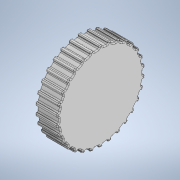
# Autodesk Inventor part: Dial_Main-Sub Menu Dial
Saved by Autodesk Inventor 2021 (Build 250183000, 183)
## iProperties
Created: 2021-05-07
Part Number: Dial_Main-Sub Menu Dial
Material: Generic
Document SubType Name: Modeling
Designer: trent
Density: 1 g/cm^3
Appearance: Default
Author: trent
Autodesk Inventor part; units mm, degrees
ref_plane "YZ Plane" through (0, 0, 0) normal (1, 0, 0) x (0, 1, 0)
ref_plane "XZ Plane" through (0, 0, 0) normal (0, 1, 0) x (-1, 0, 0)
ref_plane "XY Plane" through (0, 0, 0) normal (0, 0, 1) x (1, 0, 0)
sketch "Sketch1" plane through (0, 0, 0) normal (1, 0, 0) x (0, 1, 0)
  arc A0 (9.9984, -0.1796) -> (9.9984, 0.1796) centre (0, 0) ccw
  line L0 (0, 0) -> (11.5, 0)
  line L1 (9.7343, -0.3749) -> (9.7949, -0.376)
  line L2 (9.7343, 0.3749) -> (9.7949, 0.376)
  arc A1 (9.4805, 0.6089) -> (9.7343, 0.3749) centre (9.73, 0.6249) ccw
  arc A2 (9.7343, -0.3749) -> (9.4805, -0.6089) centre (9.73, -0.6249) ccw
  arc A3 (9.9984, 0.1796) -> (9.7949, 0.376) centre (9.7984, 0.176) ccw
  arc A4 (9.7949, -0.376) -> (9.9984, -0.1796) centre (9.7984, -0.176) ccw
  arc A5 (9.8172, 1.9031) -> (9.7426, 2.2545) centre (0, 0) ccw
  line L3 (9.5996, 1.6571) -> (9.6591, 1.6687)
  line L4 (9.4436, 2.3906) -> (9.5027, 2.4042)
  arc A6 (9.7426, 2.2545) -> (9.5027, 2.4042) centre (9.5477, 2.2094) ccw
  arc A7 (9.6591, 1.6687) -> (9.8172, 1.9031) centre (9.6209, 1.865) ccw
  arc A8 (9.1467, 2.5667) -> (9.4436, 2.3906) centre (9.3874, 2.6342) ccw
  arc A9 (9.5996, 1.6571) -> (9.3999, 1.3755) centre (9.6473, 1.4117) ccw
  arc A10 (9.207, 3.9026) -> (9.0609, 4.2308) centre (0, 0) ccw
  line L5 (9.0452, 3.6168) -> (9.101, 3.6405)
  line L6 (8.7402, 4.3018) -> (8.7952, 4.3274)
  arc A11 (9.0609, 4.2308) -> (8.7952, 4.3274) centre (8.8797, 4.1462) ccw
  arc A12 (9.101, 3.6405) -> (9.207, 3.9026) centre (9.0229, 3.8246) ccw
  arc A13 (8.4132, 4.4123) -> (8.7402, 4.3018) centre (8.6346, 4.5284) ccw
  arc A14 (9.0452, 3.6168) -> (8.9085, 3.2998) centre (9.1429, 3.3867) ccw
  arc A15 (8.1944, 5.7316) -> (7.9833, 6.0222) centre (0, 0) ccw
  line L7 (8.0956, 5.4184) -> (8.1453, 5.4531)
  line L8 (7.6549, 6.025) -> (7.7033, 6.0615)
  arc A16 (7.9833, 6.0222) -> (7.7033, 6.0615) centre (7.8236, 5.9018) ccw
  arc A17 (8.1453, 5.4531) -> (8.1944, 5.7316) centre (8.0305, 5.617) ccw
  arc A18 (7.312, 6.0651) -> (7.6549, 6.025) centre (7.5044, 6.2247) ccw
  arc A19 (8.0956, 5.4184) -> (8.0277, 5.0799) centre (8.239, 5.2136) ccw
  arc A20 (6.8237, 7.3101) -> (6.5568, 7.5504) centre (0, 0) ccw
  line L9 (6.7922, 6.9831) -> (6.8335, 7.0275)
  line L10 (6.2349, 7.4849) -> (6.2747, 7.5306)
  arc A21 (6.5568, 7.5504) -> (6.2747, 7.5306) centre (6.4256, 7.3994) ccw
  arc A22 (6.8335, 7.0275) -> (6.8237, 7.3101) centre (6.6872, 7.1639) ccw
  arc A23 (5.8912, 7.4528) -> (6.2349, 7.4849) centre (6.0462, 7.6489) ccw
  arc A24 (6.7922, 6.9831) -> (6.7961, 6.638) centre (6.975, 6.8126) ccw
  arc A25 (5.1547, 8.5691) -> (4.8436, 8.7487) centre (0, 0) ccw
  line L11 (5.1919, 8.2427) -> (5.2231, 8.2947)
  line L12 (4.5425, 8.6176) -> (4.5719, 8.6706)
  arc A26 (4.8436, 8.7487) -> (4.5719, 8.6706) centre (4.7468, 8.5737) ccw
  arc A27 (5.2231, 8.2947) -> (5.1547, 8.5691) centre (5.0516, 8.3977) ccw
  arc A28 (4.2129, 8.5148) -> (4.5425, 8.6176) centre (4.3238, 8.7388) ccw
  arc A29 (5.1919, 8.2427) -> (5.2675, 7.9059) centre (5.4061, 8.1139) ccw
  arc A30 (3.2605, 9.4535) -> (2.9189, 9.5645) centre (0, 0) ccw
  line L13 (3.3646, 9.142) -> (3.3844, 9.1993)
  line L14 (2.6515, 9.3737) -> (2.6692, 9.4317)
  arc A31 (2.9189, 9.5645) -> (2.6692, 9.4317) centre (2.8605, 9.3732) ccw
  arc A32 (3.3844, 9.1993) -> (3.2605, 9.4535) centre (3.1953, 9.2645) ccw
  arc A33 (2.3506, 9.2046) -> (2.6515, 9.3737) centre (2.4124, 9.4468) ccw
  arc A34 (3.3646, 9.142) -> (3.5087, 8.8283) centre (3.601, 9.0606) ccw
  arc A35 (1.2237, 9.9248) -> (0.8665, 9.9624) centre (0, 0) ccw
  line L15 (1.3904, 9.6418) -> (1.3978, 9.702)
  line L16 (0.6446, 9.7202) -> (0.6499, 9.7806)
  arc A36 (0.8665, 9.9624) -> (0.6499, 9.7806) centre (0.8492, 9.7631) ccw
  arc A37 (1.3978, 9.702) -> (1.2237, 9.9248) centre (1.1993, 9.7263) ccw
  arc A38 (0.3854, 9.4922) -> (0.6446, 9.7202) centre (0.3956, 9.742) ccw
  arc A39 (1.3904, 9.6418) -> (1.5965, 9.3649) centre (1.6385, 9.6113) ccw
  arc A40 (-0.8665, 9.9624) -> (-1.2237, 9.9248) centre (0, 0) ccw
  line L17 (-0.6446, 9.7202) -> (-0.6499, 9.7806)
  line L18 (-1.3904, 9.6418) -> (-1.3978, 9.702)
  arc A41 (-1.2237, 9.9248) -> (-1.3978, 9.702) centre (-1.1993, 9.7263) ccw
  arc A42 (-0.6499, 9.7806) -> (-0.8665, 9.9624) centre (-0.8492, 9.7631) ccw
  arc A43 (-1.5965, 9.3649) -> (-1.3904, 9.6418) centre (-1.6385, 9.6113) ccw
  arc A44 (-0.6446, 9.7202) -> (-0.3854, 9.4922) centre (-0.3956, 9.742) ccw
  arc A45 (-2.9189, 9.5645) -> (-3.2605, 9.4535) centre (0, 0) ccw
  line L19 (-2.6515, 9.3737) -> (-2.6692, 9.4317)
  line L20 (-3.3646, 9.142) -> (-3.3844, 9.1993)
  arc A46 (-3.2605, 9.4535) -> (-3.3844, 9.1993) centre (-3.1953, 9.2645) ccw
  arc A47 (-2.6692, 9.4317) -> (-2.9189, 9.5645) centre (-2.8605, 9.3732) ccw
  arc A48 (-3.5087, 8.8283) -> (-3.3646, 9.142) centre (-3.601, 9.0606) ccw
  arc A49 (-2.6515, 9.3737) -> (-2.3506, 9.2046) centre (-2.4124, 9.4468) ccw
  arc A50 (-4.8436, 8.7487) -> (-5.1547, 8.5691) centre (0, 0) ccw
  line L21 (-4.5425, 8.6176) -> (-4.5719, 8.6706)
  line L22 (-5.1919, 8.2427) -> (-5.2231, 8.2947)
  arc A51 (-5.1547, 8.5691) -> (-5.2231, 8.2947) centre (-5.0516, 8.3977) ccw
  arc A52 (-4.5719, 8.6706) -> (-4.8436, 8.7487) centre (-4.7468, 8.5737) ccw
  arc A53 (-5.2675, 7.9059) -> (-5.1919, 8.2427) centre (-5.4061, 8.1139) ccw
  arc A54 (-4.5425, 8.6176) -> (-4.2129, 8.5148) centre (-4.3238, 8.7388) ccw
  arc A55 (-6.5568, 7.5504) -> (-6.8237, 7.3101) centre (0, 0) ccw
  line L23 (-6.2349, 7.4849) -> (-6.2747, 7.5306)
  line L24 (-6.7922, 6.9831) -> (-6.8335, 7.0275)
  arc A56 (-6.8237, 7.3101) -> (-6.8335, 7.0275) centre (-6.6872, 7.1639) ccw
  arc A57 (-6.2747, 7.5306) -> (-6.5568, 7.5504) centre (-6.4256, 7.3994) ccw
  arc A58 (-6.7961, 6.638) -> (-6.7922, 6.9831) centre (-6.975, 6.8126) ccw
  arc A59 (-6.2349, 7.4849) -> (-5.8912, 7.4528) centre (-6.0462, 7.6489) ccw
  arc A60 (-7.9833, 6.0222) -> (-8.1944, 5.7316) centre (0, 0) ccw
  line L25 (-7.6549, 6.025) -> (-7.7033, 6.0615)
  line L26 (-8.0956, 5.4184) -> (-8.1453, 5.4531)
  arc A61 (-8.1944, 5.7316) -> (-8.1453, 5.4531) centre (-8.0305, 5.617) ccw
  arc A62 (-7.7033, 6.0615) -> (-7.9833, 6.0222) centre (-7.8236, 5.9018) ccw
  arc A63 (-8.0277, 5.0799) -> (-8.0956, 5.4184) centre (-8.239, 5.2136) ccw
  arc A64 (-7.6549, 6.025) -> (-7.312, 6.0651) centre (-7.5044, 6.2247) ccw
  arc A65 (-9.0609, 4.2308) -> (-9.207, 3.9026) centre (0, 0) ccw
  line L27 (-8.7402, 4.3018) -> (-8.7952, 4.3274)
  line L28 (-9.0452, 3.6168) -> (-9.101, 3.6405)
  arc A66 (-9.207, 3.9026) -> (-9.101, 3.6405) centre (-9.0229, 3.8246) ccw
  arc A67 (-8.7952, 4.3274) -> (-9.0609, 4.2308) centre (-8.8797, 4.1462) ccw
  arc A68 (-8.9085, 3.2998) -> (-9.0452, 3.6168) centre (-9.1429, 3.3867) ccw
  arc A69 (-8.7402, 4.3018) -> (-8.4132, 4.4123) centre (-8.6346, 4.5284) ccw
  arc A70 (-9.7426, 2.2545) -> (-9.8172, 1.9031) centre (0, 0) ccw
  line L29 (-9.4436, 2.3906) -> (-9.5027, 2.4042)
  line L30 (-9.5996, 1.6571) -> (-9.6591, 1.6687)
  arc A71 (-9.8172, 1.9031) -> (-9.6591, 1.6687) centre (-9.6209, 1.865) ccw
  arc A72 (-9.5027, 2.4042) -> (-9.7426, 2.2545) centre (-9.5477, 2.2094) ccw
  arc A73 (-9.3999, 1.3755) -> (-9.5996, 1.6571) centre (-9.6473, 1.4117) ccw
  arc A74 (-9.4436, 2.3906) -> (-9.1467, 2.5667) centre (-9.3874, 2.6342) ccw
  arc A75 (-9.9984, 0.1796) -> (-9.9984, -0.1796) centre (0, 0) ccw
  line L31 (-9.7343, 0.3749) -> (-9.7949, 0.376)
  line L32 (-9.7343, -0.3749) -> (-9.7949, -0.376)
  arc A76 (-9.9984, -0.1796) -> (-9.7949, -0.376) centre (-9.7984, -0.176) ccw
  arc A77 (-9.7949, 0.376) -> (-9.9984, 0.1796) centre (-9.7984, 0.176) ccw
  arc A78 (-9.4805, -0.6089) -> (-9.7343, -0.3749) centre (-9.73, -0.6249) ccw
  arc A79 (-9.7343, 0.3749) -> (-9.4805, 0.6089) centre (-9.73, 0.6249) ccw
  arc A80 (-9.8172, -1.9031) -> (-9.7426, -2.2545) centre (0, 0) ccw
  line L33 (-9.5996, -1.6571) -> (-9.6591, -1.6687)
  line L34 (-9.4436, -2.3906) -> (-9.5027, -2.4042)
  arc A81 (-9.7426, -2.2545) -> (-9.5027, -2.4042) centre (-9.5477, -2.2094) ccw
  arc A82 (-9.6591, -1.6687) -> (-9.8172, -1.9031) centre (-9.6209, -1.865) ccw
  arc A83 (-9.1467, -2.5667) -> (-9.4436, -2.3906) centre (-9.3874, -2.6342) ccw
  arc A84 (-9.5996, -1.6571) -> (-9.3999, -1.3755) centre (-9.6473, -1.4117) ccw
  arc A85 (-9.207, -3.9026) -> (-9.0609, -4.2308) centre (0, 0) ccw
  line L35 (-9.0452, -3.6168) -> (-9.101, -3.6405)
  line L36 (-8.7402, -4.3018) -> (-8.7952, -4.3274)
  arc A86 (-9.0609, -4.2308) -> (-8.7952, -4.3274) centre (-8.8797, -4.1462) ccw
  arc A87 (-9.101, -3.6405) -> (-9.207, -3.9026) centre (-9.0229, -3.8246) ccw
  arc A88 (-8.4132, -4.4123) -> (-8.7402, -4.3018) centre (-8.6346, -4.5284) ccw
  arc A89 (-9.0452, -3.6168) -> (-8.9085, -3.2998) centre (-9.1429, -3.3867) ccw
  arc A90 (-8.1944, -5.7316) -> (-7.9833, -6.0222) centre (0, 0) ccw
  line L37 (-8.0956, -5.4184) -> (-8.1453, -5.4531)
  line L38 (-7.6549, -6.025) -> (-7.7033, -6.0615)
  arc A91 (-7.9833, -6.0222) -> (-7.7033, -6.0615) centre (-7.8236, -5.9018) ccw
  arc A92 (-8.1453, -5.4531) -> (-8.1944, -5.7316) centre (-8.0305, -5.617) ccw
  arc A93 (-7.312, -6.0651) -> (-7.6549, -6.025) centre (-7.5044, -6.2247) ccw
  arc A94 (-8.0956, -5.4184) -> (-8.0277, -5.0799) centre (-8.239, -5.2136) ccw
  arc A95 (-6.8237, -7.3101) -> (-6.5568, -7.5504) centre (0, 0) ccw
  line L39 (-6.7922, -6.9831) -> (-6.8335, -7.0275)
  line L40 (-6.2349, -7.4849) -> (-6.2747, -7.5306)
  arc A96 (-6.5568, -7.5504) -> (-6.2747, -7.5306) centre (-6.4256, -7.3994) ccw
  arc A97 (-6.8335, -7.0275) -> (-6.8237, -7.3101) centre (-6.6872, -7.1639) ccw
  arc A98 (-5.8912, -7.4528) -> (-6.2349, -7.4849) centre (-6.0462, -7.6489) ccw
  arc A99 (-6.7922, -6.9831) -> (-6.7961, -6.638) centre (-6.975, -6.8126) ccw
  arc A100 (-5.1547, -8.5691) -> (-4.8436, -8.7487) centre (0, 0) ccw
  line L41 (-5.1919, -8.2427) -> (-5.2231, -8.2947)
  line L42 (-4.5425, -8.6176) -> (-4.5719, -8.6706)
  arc A101 (-4.8436, -8.7487) -> (-4.5719, -8.6706) centre (-4.7468, -8.5737) ccw
  arc A102 (-5.2231, -8.2947) -> (-5.1547, -8.5691) centre (-5.0516, -8.3977) ccw
  arc A103 (-4.2129, -8.5148) -> (-4.5425, -8.6176) centre (-4.3238, -8.7388) ccw
  arc A104 (-5.1919, -8.2427) -> (-5.2675, -7.9059) centre (-5.4061, -8.1139) ccw
  arc A105 (-3.2605, -9.4535) -> (-2.9189, -9.5645) centre (0, 0) ccw
  line L43 (-3.3646, -9.142) -> (-3.3844, -9.1993)
  line L44 (-2.6515, -9.3737) -> (-2.6692, -9.4317)
  arc A106 (-2.9189, -9.5645) -> (-2.6692, -9.4317) centre (-2.8605, -9.3732) ccw
  arc A107 (-3.3844, -9.1993) -> (-3.2605, -9.4535) centre (-3.1953, -9.2645) ccw
  arc A108 (-2.3506, -9.2046) -> (-2.6515, -9.3737) centre (-2.4124, -9.4468) ccw
  arc A109 (-3.3646, -9.142) -> (-3.5087, -8.8283) centre (-3.601, -9.0606) ccw
  arc A110 (-1.2237, -9.9248) -> (-0.8665, -9.9624) centre (0, 0) ccw
  line L45 (-1.3904, -9.6418) -> (-1.3978, -9.702)
  line L46 (-0.6446, -9.7202) -> (-0.6499, -9.7806)
  arc A111 (-0.8665, -9.9624) -> (-0.6499, -9.7806) centre (-0.8492, -9.7631) ccw
  arc A112 (-1.3978, -9.702) -> (-1.2237, -9.9248) centre (-1.1993, -9.7263) ccw
  arc A113 (-0.3854, -9.4922) -> (-0.6446, -9.7202) centre (-0.3956, -9.742) ccw
  arc A114 (-1.3904, -9.6418) -> (-1.5965, -9.3649) centre (-1.6385, -9.6113) ccw
  arc A115 (0.8665, -9.9624) -> (1.2237, -9.9248) centre (0, 0) ccw
  line L47 (0.6446, -9.7202) -> (0.6499, -9.7806)
  line L48 (1.3904, -9.6418) -> (1.3978, -9.702)
  arc A116 (1.2237, -9.9248) -> (1.3978, -9.702) centre (1.1993, -9.7263) ccw
  arc A117 (0.6499, -9.7806) -> (0.8665, -9.9624) centre (0.8492, -9.7631) ccw
  arc A118 (1.5965, -9.3649) -> (1.3904, -9.6418) centre (1.6385, -9.6113) ccw
  arc A119 (0.6446, -9.7202) -> (0.3854, -9.4922) centre (0.3956, -9.742) ccw
  arc A120 (2.9189, -9.5645) -> (3.2605, -9.4535) centre (0, 0) ccw
  line L49 (2.6515, -9.3737) -> (2.6692, -9.4317)
  line L50 (3.3646, -9.142) -> (3.3844, -9.1993)
  arc A121 (3.2605, -9.4535) -> (3.3844, -9.1993) centre (3.1953, -9.2645) ccw
  arc A122 (2.6692, -9.4317) -> (2.9189, -9.5645) centre (2.8605, -9.3732) ccw
  arc A123 (3.5087, -8.8283) -> (3.3646, -9.142) centre (3.601, -9.0606) ccw
  arc A124 (2.6515, -9.3737) -> (2.3506, -9.2046) centre (2.4124, -9.4468) ccw
  arc A125 (4.8436, -8.7487) -> (5.1547, -8.5691) centre (0, 0) ccw
  line L51 (4.5425, -8.6176) -> (4.5719, -8.6706)
  line L52 (5.1919, -8.2427) -> (5.2231, -8.2947)
  arc A126 (5.1547, -8.5691) -> (5.2231, -8.2947) centre (5.0516, -8.3977) ccw
  arc A127 (4.5719, -8.6706) -> (4.8436, -8.7487) centre (4.7468, -8.5737) ccw
  arc A128 (5.2675, -7.9059) -> (5.1919, -8.2427) centre (5.4061, -8.1139) ccw
  arc A129 (4.5425, -8.6176) -> (4.2129, -8.5148) centre (4.3238, -8.7388) ccw
  arc A130 (6.5568, -7.5504) -> (6.8237, -7.3101) centre (0, 0) ccw
  line L53 (6.2349, -7.4849) -> (6.2747, -7.5306)
  line L54 (6.7922, -6.9831) -> (6.8335, -7.0275)
  arc A131 (6.8237, -7.3101) -> (6.8335, -7.0275) centre (6.6872, -7.1639) ccw
  arc A132 (6.2747, -7.5306) -> (6.5568, -7.5504) centre (6.4256, -7.3994) ccw
  arc A133 (6.7961, -6.638) -> (6.7922, -6.9831) centre (6.975, -6.8126) ccw
  arc A134 (6.2349, -7.4849) -> (5.8912, -7.4528) centre (6.0462, -7.6489) ccw
  arc A135 (7.9833, -6.0222) -> (8.1944, -5.7316) centre (0, 0) ccw
  line L55 (7.6549, -6.025) -> (7.7033, -6.0615)
  line L56 (8.0956, -5.4184) -> (8.1453, -5.4531)
  arc A136 (8.1944, -5.7316) -> (8.1453, -5.4531) centre (8.0305, -5.617) ccw
  arc A137 (7.7033, -6.0615) -> (7.9833, -6.0222) centre (7.8236, -5.9018) ccw
  arc A138 (8.0277, -5.0799) -> (8.0956, -5.4184) centre (8.239, -5.2136) ccw
  arc A139 (7.6549, -6.025) -> (7.312, -6.0651) centre (7.5044, -6.2247) ccw
  arc A140 (9.0609, -4.2308) -> (9.207, -3.9026) centre (0, 0) ccw
  line L57 (8.7402, -4.3018) -> (8.7952, -4.3274)
  line L58 (9.0452, -3.6168) -> (9.101, -3.6405)
  arc A141 (9.207, -3.9026) -> (9.101, -3.6405) centre (9.0229, -3.8246) ccw
  arc A142 (8.7952, -4.3274) -> (9.0609, -4.2308) centre (8.8797, -4.1462) ccw
  arc A143 (8.9085, -3.2998) -> (9.0452, -3.6168) centre (9.1429, -3.3867) ccw
  arc A144 (8.7402, -4.3018) -> (8.4132, -4.4123) centre (8.6346, -4.5284) ccw
  arc A145 (9.7426, -2.2545) -> (9.8172, -1.9031) centre (0, 0) ccw
  line L59 (9.4436, -2.3906) -> (9.5027, -2.4042)
  line L60 (9.5996, -1.6571) -> (9.6591, -1.6687)
  arc A146 (9.8172, -1.9031) -> (9.6591, -1.6687) centre (9.6209, -1.865) ccw
  arc A147 (9.5027, -2.4042) -> (9.7426, -2.2545) centre (9.5477, -2.2094) ccw
  arc A148 (9.3999, -1.3755) -> (9.5996, -1.6571) centre (9.6473, -1.4117) ccw
  arc A149 (9.4436, -2.3906) -> (9.1467, -2.5667) centre (9.3874, -2.6342) ccw
  arc A150 (9.3999, -1.3755) -> (9.4805, -0.6089) centre (0, 0) ccw
  arc A151 (8.9085, -3.2998) -> (9.1467, -2.5667) centre (0, 0) ccw
  arc A152 (8.0277, -5.0799) -> (8.4132, -4.4123) centre (0, 0) ccw
  arc A153 (6.7961, -6.638) -> (7.312, -6.0651) centre (0, 0) ccw
  arc A154 (5.2675, -7.9059) -> (5.8912, -7.4528) centre (0, 0) ccw
  arc A155 (3.5087, -8.8283) -> (4.2129, -8.5148) centre (0, 0) ccw
  arc A156 (1.5965, -9.3649) -> (2.3506, -9.2046) centre (0, 0) ccw
  arc A157 (-0.3854, -9.4922) -> (0.3854, -9.4922) centre (0, 0) ccw
  arc A158 (-2.3506, -9.2046) -> (-1.5965, -9.3649) centre (0, 0) ccw
  arc A159 (-4.2129, -8.5148) -> (-3.5087, -8.8283) centre (0, 0) ccw
  arc A160 (-5.8912, -7.4528) -> (-5.2675, -7.9059) centre (0, 0) ccw
  arc A161 (-7.312, -6.0651) -> (-6.7961, -6.638) centre (0, 0) ccw
  arc A162 (-8.4132, -4.4123) -> (-8.0277, -5.0799) centre (0, 0) ccw
  arc A163 (-9.1467, -2.5667) -> (-8.9085, -3.2998) centre (0, 0) ccw
  arc A164 (-9.4805, -0.6089) -> (-9.3999, -1.3755) centre (0, 0) ccw
  arc A165 (-9.3999, 1.3755) -> (-9.4805, 0.6089) centre (0, 0) ccw
  arc A166 (-8.9085, 3.2998) -> (-9.1467, 2.5667) centre (0, 0) ccw
  arc A167 (-8.0277, 5.0799) -> (-8.4132, 4.4123) centre (0, 0) ccw
  arc A168 (-6.7961, 6.638) -> (-7.312, 6.0651) centre (0, 0) ccw
  arc A169 (-5.2675, 7.9059) -> (-5.8912, 7.4528) centre (0, 0) ccw
  arc A170 (-3.5087, 8.8283) -> (-4.2129, 8.5148) centre (0, 0) ccw
  arc A171 (-1.5965, 9.3649) -> (-2.3506, 9.2046) centre (0, 0) ccw
  arc A172 (0.3854, 9.4922) -> (-0.3854, 9.4922) centre (0, 0) ccw
  arc A173 (2.3506, 9.2046) -> (1.5965, 9.3649) centre (0, 0) ccw
  arc A174 (4.2129, 8.5148) -> (3.5087, 8.8283) centre (0, 0) ccw
  arc A175 (5.8912, 7.4528) -> (5.2675, 7.9059) centre (0, 0) ccw
  arc A176 (7.312, 6.0651) -> (6.7961, 6.638) centre (0, 0) ccw
  arc A177 (8.4132, 4.4123) -> (8.0277, 5.0799) centre (0, 0) ccw
  arc A178 (9.4805, 0.6089) -> (9.3999, 1.3755) centre (0, 0) ccw
  arc A179 (9.1467, 2.5667) -> (8.9085, 3.2998) centre (0, 0) ccw
  point P0 (9.9928, -0.3794)
  point P1 (9.9928, 0.3794)
  point P2 (11.4928, 0.4056)
  point P3 (11.4928, -0.4056)
  dimension "d1" = 20
  dimension "d2" = 1
  dimension "d3" = 1
  dimension "d4" = 0.25
  dimension "d5" = 0.2
  dimension "d8" = 360
  dimension "d14" = 0.41
  dimension "d15" = 0.41
  dimension "d16" = 0.4057
  dimension "d17" = 0.8111
  dimension "d18" = 2.3861
  constraints: 302 point on circle, 150 centre point, 122 end point, 122 equal radius, 60 equal length, 30 coincident, 30 concentric, 8 tangent, 4 point on line, 2 horizontal alignment, 1 horizontal, 451 other
  measures "d1" diameter of A0
  measures "d2" angle of L2 L0
  measures "d3" angle of L1 L0
  measures "d4" radius of A1
  measures "d5" radius of A3
  measures "d14" distance between parallel lines of L1 L31
  measures "d15" distance between parallel lines of L2 L32
  measures "d16" distance from line of L0.end L1
  measures "d17" distance from line of point (11.493, 0.406) L1
  measures "d18" distance from line of point (11.493, -0.406) L3
extrude "Extrusion1" add sketch "Sketch1" along normal blind 5
fillet "Fillet1" radius 0.25 240 edges at (0, 9.5605, 0.441) (0, 9.448, 0.993) (0, 9.4433, 1.5563) (0, 9.6293, 1.6629) (0, 9.7867, 1.7532) (0, 9.7815, 2.0791) (0, 9.6536, 2.379) (0, 9.4732, 2.3974) (0, 9.2599, 2.4192) (0, 9.035, 2.9357) (0, 8.9134, 3.4857) (0, 9.0731, 3.6286) (0, 9.2083, 3.7496) (0, 9.1355, 4.0674) (0, 8.9481, 4.3341) (0, 8.7677, 4.3146) (0, 8.5546, 4.2915) (0, 8.2272, 4.75) (0, 7.9939, 5.2627) (0, 8.1204, 5.4358) (0, 8.2275, 5.5822) (0, 8.0902, 5.8779) (0, 7.8514, 6.0998) (0, 7.6791, 6.0433) (0, 7.4754, 5.9764) (0, 7.0599, 6.3567) (0, 6.725, 6.8097) (0, 6.8128, 7.0053) (0, 6.8871, 7.1708) (0, 6.6913, 7.4314) (0, 6.4116, 7.5989) (0, 6.2548, 7.5078) (0, 6.0695, 7.4) (0, 5.584, 7.6857) (0, 5.1622, 8.0591) (0, 5.2075, 8.2687) (0, 5.2457, 8.446) (0, 5, 8.6603) (0, 4.6916, 8.7659) (0, 4.5572, 8.6441) (0, 4.3983, 8.5002) (0, 3.864, 8.6787) (0, 3.3738, 8.9563) (0, 3.3745, 9.1707) (0, 3.3751, 9.3521) (0, 3.0902, 9.5106) (0, 2.7665, 9.5498) (0, 2.6604, 9.4027) (0, 2.5349, 9.2289) (0, 1.9752, 9.2924) (0, 1.438, 9.4621) (0, 1.3941, 9.6719) (0, 1.3569, 9.8494) (0, 1.0453, 9.9452) (0, 0.7206, 9.9163) (0, 0.6473, 9.7504) (0, 0.5607, 9.5543) (0, 0, 9.5) (0, -0.5607, 9.5543) (0, -0.6473, 9.7504) (0, -0.7206, 9.9163) (0, -1.0453, 9.9452) (0, -1.3569, 9.8494) (0, -1.3941, 9.6719) (0, -1.438, 9.4621) (0, -1.9752, 9.2924) (0, -2.5349, 9.2289) (0, -2.6604, 9.4027) (0, -2.7665, 9.5498) (0, -3.0902, 9.5106) (0, -3.3751, 9.3521) (0, -3.3745, 9.1707) (0, -3.3738, 8.9563) (0, -3.864, 8.6787) (0, -4.3983, 8.5002) (0, -4.5572, 8.6441) (0, -4.6916, 8.7659) (0, -5, 8.6603) (0, -5.2457, 8.446) (0, -5.2075, 8.2687) (0, -5.1622, 8.0591) (0, -5.584, 7.6857) (0, -6.0695, 7.4) (0, -6.2548, 7.5078) (0, -6.4116, 7.5989) (0, -6.6913, 7.4314) (0, -6.8871, 7.1708) (0, -6.8128, 7.0053) (0, -6.725, 6.8097) (0, -7.0599, 6.3567) (0, -7.4754, 5.9764) (0, -7.6791, 6.0433) (0, -7.8514, 6.0998) (0, -8.0902, 5.8779) (0, -8.2275, 5.5822) (0, -8.1204, 5.4358) (0, -7.9939, 5.2627) (0, -8.2272, 4.75) (0, -8.5546, 4.2915) (0, -8.7677, 4.3146) (0, -8.9481, 4.3341) (0, -9.1355, 4.0674) (0, -9.2083, 3.7496) (0, -9.0731, 3.6286) (0, -8.9134, 3.4857) (0, -9.035, 2.9357) (0, -9.2599, 2.4192) (0, -9.4732, 2.3974) (0, -9.6536, 2.379) (0, -9.7815, 2.0791) (0, -9.7867, 1.7532) (0, -9.6293, 1.6629) (0, -9.4433, 1.5563) (0, -9.448, 0.993) (0, -9.5605, 0.441) (0, -9.7646, 0.3755) (0, -9.9373, 0.3199) (0, -10, 0) (0, -9.9373, -0.3199) (0, -9.7646, -0.3755) (0, -9.5605, -0.441) (0, -9.448, -0.993) (0, -9.4433, -1.5563) (0, -9.6293, -1.6629) (0, -9.7867, -1.7532) (0, -9.7815, -2.0791) (0, -9.6536, -2.379) (0, -9.4732, -2.3974) (0, -9.2599, -2.4192) (0, -9.035, -2.9357) (0, -8.9134, -3.4857) (0, -9.0731, -3.6286) (0, -9.2083, -3.7496) (0, -9.1355, -4.0674) (0, -8.9481, -4.3341) (0, -8.7677, -4.3146) (0, -8.5546, -4.2915) (0, -8.2272, -4.75) (0, -7.9939, -5.2627) (0, -8.1204, -5.4358) (0, -8.2275, -5.5822) (0, -8.0902, -5.8779) (0, -7.8514, -6.0998) (0, -7.6791, -6.0433) (0, -7.4754, -5.9764) (0, -7.0599, -6.3567) (0, -6.725, -6.8097) (0, -6.8128, -7.0053) (0, -6.8871, -7.1708) (0, -6.6913, -7.4314) (0, -6.4116, -7.5989) (0, -6.2548, -7.5078) (0, -6.0695, -7.4) (0, -5.584, -7.6857) (0, -5.1622, -8.0591) (0, -5.2075, -8.2687) (0, -5.2457, -8.446) (0, -5, -8.6603) (0, -4.6916, -8.7659) (0, -4.5572, -8.6441) (0, -4.3983, -8.5002) (0, -3.864, -8.6787) (0, -3.3738, -8.9563) (0, -3.3745, -9.1707) (0, -3.3751, -9.3521) (0, -3.0902, -9.5106) (0, -2.7665, -9.5498) (0, -2.6604, -9.4027) (0, -2.5349, -9.2289) (0, -1.9752, -9.2924) (0, -1.438, -9.4621) (0, -1.3941, -9.6719) (0, -1.3569, -9.8494) (0, -1.0453, -9.9452) (0, -0.7206, -9.9163) (0, -0.6473, -9.7504) (0, -0.5607, -9.5543) (0, 0, -9.5) (0, 0.5607, -9.5543) (0, 0.6473, -9.7504) (0, 0.7206, -9.9163) (0, 1.0453, -9.9452) (0, 1.3569, -9.8494) (0, 1.3941, -9.6719) (0, 1.438, -9.4621) (0, 1.9752, -9.2924) (0, 2.5349, -9.2289) (0, 2.6604, -9.4027) (0, 2.7665, -9.5498) (0, 3.0902, -9.5106) (0, 3.3751, -9.3521) (0, 3.3745, -9.1707) (0, 3.3738, -8.9563) (0, 3.864, -8.6787) (0, 4.3983, -8.5002) (0, 4.5572, -8.6441) (0, 4.6916, -8.7659) (0, 5, -8.6603) (0, 5.2457, -8.446) (0, 5.2075, -8.2687) (0, 5.1622, -8.0591) (0, 5.584, -7.6857) (0, 6.0695, -7.4) (0, 6.2548, -7.5078) (0, 6.4116, -7.5989) (0, 6.6913, -7.4314) (0, 6.8871, -7.1708) (0, 6.8128, -7.0053) (0, 6.725, -6.8097) (0, 7.0599, -6.3567) (0, 7.4754, -5.9764) (0, 7.6791, -6.0433) (0, 7.8514, -6.0998) (0, 8.0902, -5.8779) (0, 8.2275, -5.5822) (0, 8.1204, -5.4358) (0, 7.9939, -5.2627) (0, 8.2272, -4.75) (0, 8.5546, -4.2915) (0, 8.7677, -4.3146) (0, 8.9481, -4.3341) (0, 9.1355, -4.0674) (0, 9.2083, -3.7496) (0, 9.0731, -3.6286) (0, 8.9134, -3.4857) (0, 9.035, -2.9357) (0, 9.2599, -2.4192) (0, 9.4732, -2.3974) (0, 9.6536, -2.379) (0, 9.7815, -2.0791) (0, 9.7867, -1.7532) (0, 9.6293, -1.6629) (0, 9.4433, -1.5563) (0, 9.448, -0.993) (0, 9.5605, -0.441) (0, 9.7646, -0.3755) (0, 9.9373, -0.3199) (0, 10, 0) (0, 9.9373, 0.3199) (0, 9.7646, 0.3755)
fillet "Fillet2" radius 0.25 240 edges at (5, 7.8514, 6.0998) (5, 7.6791, 6.0433) (5, 7.4754, 5.9764) (5, 7.0599, 6.3567) (5, 6.725, 6.8097) (5, 6.8128, 7.0053) (5, 6.8871, 7.1708) (5, 6.6913, 7.4314) (5, 6.4116, 7.5989) (5, 6.2548, 7.5078) (5, 6.0695, 7.4) (5, 5.584, 7.6857) (5, 5.1622, 8.0591) (5, 5.2075, 8.2687) (5, 5.2457, 8.446) (5, 5, 8.6603) (5, 4.6916, 8.7659) (5, 4.5572, 8.6441) (5, 4.3983, 8.5002) (5, 3.864, 8.6787) (5, 3.3738, 8.9563) (5, 3.3745, 9.1707) (5, 3.3751, 9.3521) (5, 3.0902, 9.5106) (5, 2.7665, 9.5498) (5, 2.6604, 9.4027) (5, 2.5349, 9.2289) (5, 1.9752, 9.2924) (5, 1.438, 9.4621) (5, 1.3941, 9.6719) (5, 1.3569, 9.8494) (5, 1.0453, 9.9452) (5, 0.7206, 9.9163) (5, 0.6473, 9.7504) (5, 0.5607, 9.5543) (5, 0, 9.5) (5, -0.5607, 9.5543) (5, -0.6473, 9.7504) (5, -0.7206, 9.9163) (5, -1.0453, 9.9452) (5, -1.3569, 9.8494) (5, -1.3941, 9.6719) (5, -1.438, 9.4621) (5, -1.9752, 9.2924) (5, -2.5349, 9.2289) (5, -2.6604, 9.4027) (5, -2.7665, 9.5498) (5, -3.0902, 9.5106) (5, -3.3751, 9.3521) (5, -3.3745, 9.1707) (5, -3.3738, 8.9563) (5, -3.864, 8.6787) (5, -4.3983, 8.5002) (5, -4.5572, 8.6441) (5, -4.6916, 8.7659) (5, -5, 8.6603) (5, -5.2457, 8.446) (5, -5.2075, 8.2687) (5, -5.1622, 8.0591) (5, -5.584, 7.6857) (5, -6.0695, 7.4) (5, -6.2548, 7.5078) (5, -6.4116, 7.5989) (5, -6.6913, 7.4314) (5, -6.8871, 7.1708) (5, -6.8128, 7.0053) (5, -6.725, 6.8097) (5, -7.0599, 6.3567) (5, -7.4754, 5.9764) (5, -7.6791, 6.0433) (5, -7.8514, 6.0998) (5, -8.0902, 5.8779) (5, -8.2275, 5.5822) (5, -8.1204, 5.4358) (5, -7.9939, 5.2627) (5, -8.2272, 4.75) (5, -8.5546, 4.2915) (5, -8.7677, 4.3146) (5, -8.9481, 4.3341) (5, -9.1355, 4.0674) (5, -9.2083, 3.7496) (5, -9.0731, 3.6286) (5, -8.9134, 3.4857) (5, -9.035, 2.9357) (5, -9.2599, 2.4192) (5, -9.4732, 2.3974) (5, -9.6536, 2.379) (5, -9.7815, 2.0791) (5, -9.7867, 1.7532) (5, -9.6293, 1.6629) (5, -9.4433, 1.5563) (5, -9.448, 0.993) (5, -9.5605, 0.441) (5, -9.7646, 0.3755) (5, -9.9373, 0.3199) (5, -10, 0) (5, -9.9373, -0.3199) (5, -9.7646, -0.3755) (5, -9.5605, -0.441) (5, -9.448, -0.993) (5, -9.4433, -1.5563) (5, -9.6293, -1.6629) (5, -9.7867, -1.7532) (5, -9.7815, -2.0791) (5, -9.6536, -2.379) (5, -9.4732, -2.3974) (5, -9.2599, -2.4192) (5, -9.035, -2.9357) (5, -8.9134, -3.4857) (5, -9.0731, -3.6286) (5, -9.2083, -3.7496) (5, -9.1355, -4.0674) (5, -8.9481, -4.3341) (5, -8.7677, -4.3146) (5, -8.5546, -4.2915) (5, -8.2272, -4.75) (5, -7.9939, -5.2627) (5, -8.1204, -5.4358) (5, -8.2275, -5.5822) (5, -8.0902, -5.8779) (5, -7.8514, -6.0998) (5, -7.6791, -6.0433) (5, -7.4754, -5.9764) (5, -7.0599, -6.3567) (5, -6.725, -6.8097) (5, -6.8128, -7.0053) (5, -6.8871, -7.1708) (5, -6.6913, -7.4314) (5, -6.4116, -7.5989) (5, -6.2548, -7.5078) (5, -6.0695, -7.4) (5, -5.584, -7.6857) (5, -5.1622, -8.0591) (5, -5.2075, -8.2687) (5, -5.2457, -8.446) (5, -5, -8.6603) (5, -4.6916, -8.7659) (5, -4.5572, -8.6441) (5, -4.3983, -8.5002) (5, -3.864, -8.6787) (5, -3.3738, -8.9563) (5, -3.3745, -9.1707) (5, -3.3751, -9.3521) (5, -3.0902, -9.5106) (5, -2.7665, -9.5498) (5, -2.6604, -9.4027) (5, -2.5349, -9.2289) (5, -1.9752, -9.2924) (5, -1.438, -9.4621) (5, -1.3941, -9.6719) (5, -1.3569, -9.8494) (5, -1.0453, -9.9452) (5, -0.7206, -9.9163) (5, -0.6473, -9.7504) (5, -0.5607, -9.5543) (5, 0, -9.5) (5, 0.5607, -9.5543) (5, 0.6473, -9.7504) (5, 0.7206, -9.9163) (5, 1.0453, -9.9452) (5, 1.3569, -9.8494) (5, 1.3941, -9.6719) (5, 1.438, -9.4621) (5, 1.9752, -9.2924) (5, 2.5349, -9.2289) (5, 2.6604, -9.4027) (5, 2.7665, -9.5498) (5, 3.0902, -9.5106) (5, 3.3751, -9.3521) (5, 3.3745, -9.1707) (5, 3.3738, -8.9563) (5, 3.864, -8.6787) (5, 4.3983, -8.5002) (5, 4.5572, -8.6441) (5, 4.6916, -8.7659) (5, 5, -8.6603) (5, 5.2457, -8.446) (5, 5.2075, -8.2687) (5, 5.1622, -8.0591) (5, 5.584, -7.6857) (5, 6.0695, -7.4) (5, 6.2548, -7.5078) (5, 6.4116, -7.5989) (5, 6.6913, -7.4314) (5, 6.8871, -7.1708) (5, 6.8128, -7.0053) (5, 6.725, -6.8097) (5, 7.0599, -6.3567) (5, 7.4754, -5.9764) (5, 7.6791, -6.0433) (5, 7.8514, -6.0998) (5, 8.0902, -5.8779) (5, 8.2275, -5.5822) (5, 8.1204, -5.4358) (5, 7.9939, -5.2627) (5, 8.2272, -4.75) (5, 8.5546, -4.2915) (5, 8.7677, -4.3146) (5, 8.9481, -4.3341) (5, 9.1355, -4.0674) (5, 9.2083, -3.7496) (5, 9.0731, -3.6286) (5, 8.9134, -3.4857) (5, 9.035, -2.9357) (5, 9.2599, -2.4192) (5, 9.4732, -2.3974) (5, 9.6536, -2.379) (5, 9.7815, -2.0791) (5, 9.7867, -1.7532) (5, 9.6293, -1.6629) (5, 9.4433, -1.5563) (5, 9.448, -0.993) (5, 9.5605, -0.441) (5, 9.7646, -0.3755) (5, 9.9373, -0.3199) (5, 10, 0) (5, 9.9373, 0.3199) (5, 9.7646, 0.3755) (5, 9.5605, 0.441) (5, 9.448, 0.993) (5, 9.4433, 1.5563) (5, 9.6293, 1.6629) (5, 9.7867, 1.7532) (5, 9.7815, 2.0791) (5, 9.6536, 2.379) (5, 9.4732, 2.3974) (5, 9.2599, 2.4192) (5, 9.035, 2.9357) (5, 8.9134, 3.4857) (5, 9.0731, 3.6286) (5, 9.2083, 3.7496) (5, 9.1355, 4.0674) (5, 8.9481, 4.3341) (5, 8.7677, 4.3146) (5, 8.5546, 4.2915) (5, 8.2272, 4.75) (5, 7.9939, 5.2627) (5, 8.1204, 5.4358) (5, 8.2275, 5.5822) (5, 8.0902, 5.8779)
equation "\"d3\" = d2"
body "Solid1"
